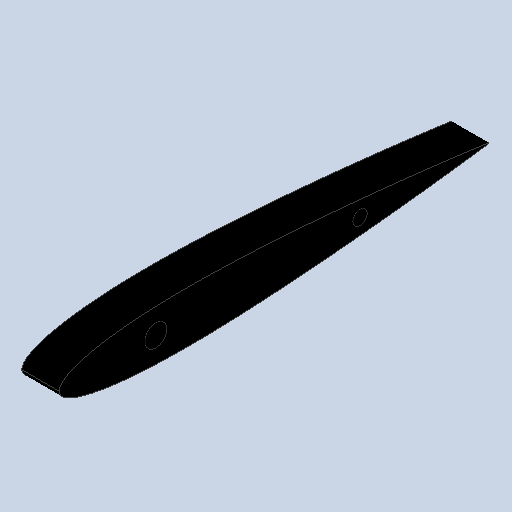
# Autodesk Inventor part: 6P-009
Saved by Autodesk Inventor 2025.2 (Build 292293000, 293)
## iProperties
Category: <PART CATAGORY>
Created: 2024-11-15
Part Number: 6P-009
Material: Poplar
Document SubType Name: Modeling
Designer: lachl
Density: 0.448 g/cm^3
Appearance: Default
Mass: 2.73512 g
Surface Area: 51.8943 cm^2
Volume: 6.10518 cm^3
Title: <TITLE>
Author: lachl
Revision Number: 1
Autodesk Inventor part; units mm, degrees
ref_plane "YZ Plane" through (0, 0, 0) normal (1, 0, 0) x (0, 1, 0)
ref_plane "XZ Plane" through (0, 0, 0) normal (0, 1, 0) x (-1, 0, 0)
ref_plane "XY Plane" through (0, 0, 0) normal (0, 0, 1) x (1, 0, 0)
sketch "Sketch9" plane through (0, 0, 0) normal (1, 0, 0) x (0, 1, 0)
  line L0 (0, 0) -> (0.6838, -0.0937) construction
  line L1 (0.6838, -0.0937) -> (1.3528, -0.3746) construction
  line L2 (1.3528, -0.3746) -> (2.0064, -0.8421) construction
  line L3 (2.0064, -0.8421) -> (2.6435, -1.495) construction
  line L4 (2.6435, -1.495) -> (3.263, -2.3319) construction
  line L5 (3.263, -2.3319) -> (3.8633, -3.3508) construction
  line L6 (3.8633, -3.3508) -> (4.4431, -4.5492) construction
  line L7 (4.4431, -4.5492) -> (5.0005, -5.9245) construction
  line L8 (5.0005, -5.9245) -> (5.5339, -7.4733) construction
  line L9 (5.5339, -7.4733) -> (6.0414, -9.1922) construction
  line L10 (6.0414, -9.1922) -> (6.5213, -11.0769) construction
  line L11 (6.5213, -11.0769) -> (6.9717, -13.1233) construction
  line L12 (6.9717, -13.1233) -> (7.3908, -15.3264) construction
  line L13 (7.3908, -15.3264) -> (7.7773, -17.6811) construction
  line L14 (7.7773, -17.6811) -> (8.1295, -20.182) construction
  line L15 (8.1295, -20.182) -> (8.4463, -22.8232) construction
  line L16 (8.4463, -22.8232) -> (8.7266, -25.5985) construction
  line L17 (8.7266, -25.5985) -> (8.9696, -28.5014) construction
  line L18 (8.9696, -28.5014) -> (9.1748, -31.5252) construction
  line L19 (9.1748, -31.5252) -> (9.3419, -34.6628) construction
  line L20 (9.3419, -34.6628) -> (9.4708, -37.9069) construction
  line L21 (9.4708, -37.9069) -> (9.5619, -41.2498) construction
  line L22 (9.5619, -41.2498) -> (9.6156, -44.6839) construction
  line L23 (9.6156, -44.6839) -> (9.6156, -48.201) construction
  line L24 (9.6156, -48.201) -> (9.6156, -51.793) construction
  line L25 (9.6156, -51.793) -> (9.5617, -55.4514) construction
  line L26 (9.5617, -55.4514) -> (9.4762, -59.1677) construction
  line L27 (9.4762, -59.1677) -> (9.3595, -62.9333) construction
  line L28 (9.3595, -62.9333) -> (9.2132, -66.7394) construction
  line L29 (9.2132, -66.7394) -> (9.0394, -70.5769) construction
  line L30 (9.0394, -70.5769) -> (8.8398, -74.4371) construction
  line L31 (8.8398, -74.4371) -> (8.6167, -78.3109) construction
  line L32 (8.6167, -78.3109) -> (8.372, -82.1891) construction
  line L33 (8.372, -82.1891) -> (8.1078, -86.0629) construction
  line L34 (8.1078, -86.0629) -> (7.8263, -89.9231) construction
  line L35 (7.8263, -89.9231) -> (7.5294, -93.7607) construction
  line L36 (7.5294, -93.7607) -> (7.2193, -97.5667) construction
  line L37 (7.2193, -97.5667) -> (6.8979, -101.3323) construction
  line L38 (6.8979, -101.3323) -> (6.5672, -105.0486) construction
  line L39 (6.5672, -105.0486) -> (6.2291, -108.7071) construction
  line L40 (6.2291, -108.7071) -> (5.8855, -112.299) construction
  line L41 (5.8855, -112.299) -> (5.5382, -115.8161) construction
  line L42 (5.5382, -115.8161) -> (5.1889, -119.2502) construction
  line L43 (5.1889, -119.2502) -> (4.8393, -122.5931) construction
  line L44 (4.8393, -122.5931) -> (4.4912, -125.8372) construction
  line L45 (4.4912, -125.8372) -> (4.1463, -128.9748) construction
  line L46 (4.1463, -128.9748) -> (3.8061, -131.9986) construction
  line L47 (3.8061, -131.9986) -> (3.4724, -134.9015) construction
  line L48 (3.4724, -134.9015) -> (3.1466, -137.6768) construction
  line L49 (3.1466, -137.6768) -> (2.8305, -140.318) construction
  line L50 (2.8305, -140.318) -> (2.5255, -142.8189) construction
  line L51 (2.5255, -142.8189) -> (2.2332, -145.1736) construction
  line L52 (2.2332, -145.1736) -> (1.9553, -147.3767) construction
  line L53 (1.9553, -147.3767) -> (1.693, -149.4231) construction
  line L54 (1.693, -149.4231) -> (1.448, -151.3078) construction
  line L55 (1.448, -151.3078) -> (1.2215, -153.0267) construction
  line L56 (1.2215, -153.0267) -> (1.015, -154.5755) construction
  line L57 (1.015, -154.5755) -> (0.8295, -155.9508) construction
  line L58 (0.8295, -155.9508) -> (0.6664, -157.1492) construction
  line L59 (0.6664, -157.1492) -> (0.5265, -158.1681) construction
  line L60 (0.5265, -158.1681) -> (0.4108, -159.0049) construction
  line L61 (0.4108, -159.0049) -> (0.32, -159.6579) construction
  line L62 (0.32, -159.6579) -> (0.2547, -160.1254) construction
  line L63 (0.2547, -160.1254) -> (0.2154, -160.4063) construction
  line L64 (0.2154, -160.4063) -> (0.2022, -160.5) construction
  line L65 (0.2022, -160.5) -> (0, -161.463) construction
  line L66 (0, -161.463) -> (-0.2022, -160.5) construction
  line L67 (-0.2022, -160.5) -> (-0.2154, -160.4063) construction
  line L68 (-0.2154, -160.4063) -> (-0.2547, -160.1254) construction
  line L69 (-0.2547, -160.1254) -> (-0.32, -159.6579) construction
  line L70 (-0.32, -159.6579) -> (-0.4108, -159.0049) construction
  line L71 (-0.4108, -159.0049) -> (-0.5265, -158.1681) construction
  line L72 (-0.5265, -158.1681) -> (-0.6664, -157.1492) construction
  line L73 (-0.6664, -157.1492) -> (-0.8295, -155.9508) construction
  line L74 (-0.8295, -155.9508) -> (-1.015, -154.5755) construction
  line L75 (-1.015, -154.5755) -> (-1.2215, -153.0267) construction
  line L76 (-1.2215, -153.0267) -> (-1.448, -151.3078) construction
  line L77 (-1.448, -151.3078) -> (-1.693, -149.4231) construction
  line L78 (-1.693, -149.4231) -> (-1.9553, -147.3767) construction
  line L79 (-1.9553, -147.3767) -> (-2.2332, -145.1736) construction
  line L80 (-2.2332, -145.1736) -> (-2.5255, -142.8189) construction
  line L81 (-2.5255, -142.8189) -> (-2.8305, -140.318) construction
  line L82 (-2.8305, -140.318) -> (-3.1466, -137.6768) construction
  line L83 (-3.1466, -137.6768) -> (-3.4724, -134.9015) construction
  line L84 (-3.4724, -134.9015) -> (-3.8061, -131.9986) construction
  line L85 (-3.8061, -131.9986) -> (-4.1463, -128.9748) construction
  line L86 (-4.1463, -128.9748) -> (-4.4912, -125.8372) construction
  line L87 (-4.4912, -125.8372) -> (-4.8393, -122.5931) construction
  line L88 (-4.8393, -122.5931) -> (-5.1889, -119.2502) construction
  line L89 (-5.1889, -119.2502) -> (-5.5382, -115.8161) construction
  line L90 (-5.5382, -115.8161) -> (-5.8855, -112.299) construction
  line L91 (-5.8855, -112.299) -> (-6.2291, -108.7071) construction
  line L92 (-6.2291, -108.7071) -> (-6.5672, -105.0486) construction
  line L93 (-6.5672, -105.0486) -> (-6.8979, -101.3323) construction
  line L94 (-6.8979, -101.3323) -> (-7.2193, -97.5667) construction
  line L95 (-7.2193, -97.5667) -> (-7.5294, -93.7607) construction
  line L96 (-7.5294, -93.7607) -> (-7.8263, -89.9231) construction
  line L97 (-7.8263, -89.9231) -> (-8.1078, -86.0629) construction
  line L98 (-8.1078, -86.0629) -> (-8.372, -82.1891) construction
  line L99 (-8.372, -82.1891) -> (-8.6167, -78.3109) construction
  line L100 (-8.6167, -78.3109) -> (-8.8398, -74.4371) construction
  line L101 (-8.8398, -74.4371) -> (-9.0394, -70.5769) construction
  line L102 (-9.0394, -70.5769) -> (-9.2132, -66.7394) construction
  line L103 (-9.2132, -66.7394) -> (-9.3595, -62.9333) construction
  line L104 (-9.3595, -62.9333) -> (-9.4762, -59.1677) construction
  line L105 (-9.4762, -59.1677) -> (-9.5617, -55.4514) construction
  line L106 (-9.5617, -55.4514) -> (-9.6144, -51.793) construction
  line L107 (-9.6144, -51.793) -> (-9.6144, -48.201) construction
  line L108 (-9.6144, -48.201) -> (-9.6144, -44.6839) construction
  line L109 (-9.6144, -44.6839) -> (-9.5619, -41.2498) construction
  line L110 (-9.5619, -41.2498) -> (-9.4708, -37.9069) construction
  line L111 (-9.4708, -37.9069) -> (-9.3419, -34.6628) construction
  line L112 (-9.3419, -34.6628) -> (-9.1748, -31.5252) construction
  line L113 (-9.1748, -31.5252) -> (-8.9696, -28.5014) construction
  line L114 (-8.9696, -28.5014) -> (-8.7266, -25.5985) construction
  line L115 (-8.7266, -25.5985) -> (-8.4463, -22.8232) construction
  line L116 (-8.4463, -22.8232) -> (-8.1295, -20.182) construction
  line L117 (-8.1295, -20.182) -> (-7.7773, -17.6811) construction
  line L118 (-7.7773, -17.6811) -> (-7.3908, -15.3264) construction
  line L119 (-7.3908, -15.3264) -> (-6.9717, -13.1233) construction
  line L120 (-6.9717, -13.1233) -> (-6.5213, -11.0769) construction
  line L121 (-6.5213, -11.0769) -> (-6.0414, -9.1922) construction
  line L122 (-6.0414, -9.1922) -> (-5.5339, -7.4733) construction
  line L123 (-5.5339, -7.4733) -> (-5.0005, -5.9245) construction
  line L124 (-5.0005, -5.9245) -> (-4.4431, -4.5492) construction
  line L125 (-4.4431, -4.5492) -> (-3.8633, -3.3508) construction
  line L126 (-3.8633, -3.3508) -> (-3.263, -2.3319) construction
  line L127 (-3.263, -2.3319) -> (-2.6435, -1.495) construction
  line L128 (-2.6435, -1.495) -> (-2.0064, -0.8421) construction
  line L129 (-2.0064, -0.8421) -> (-1.3528, -0.3746) construction
  line L130 (-1.3528, -0.3746) -> (-0.6838, -0.0937) construction
  line L131 (-0.6838, -0.0937) -> (0, 0) construction
  spline S0 degree 4 poles (0, 0) (0.6838, -0.0937) (1.3528, -0.3746) (2.0064, -0.8421) (2.6435, -1.495) (3.263, -2.3319) (3.8633, -3.3508) (4.4431, -4.5492) (5.0005, -5.9245) (5.5339, -7.4733) (6.0414, -9.1922) (6.5213, -11.0769) (6.9717, -13.1233) (7.3908, -15.3264) (7.7773, -17.6811) (8.1295, -20.182) (8.4463, -22.8232) (8.7266, -25.5985) (8.9696, -28.5014) (9.1748, -31.5252) (9.3419, -34.6628) (9.4708, -37.9069) (9.5619, -41.2498) (9.6156, -44.6839) (9.6156, -48.201) (9.6156, -51.793) (9.5617, -55.4514) (9.4762, -59.1677) (9.3595, -62.9333) (9.2132, -66.7394) (9.0394, -70.5769) (8.8398, -74.4371) (8.6167, -78.3109) (8.372, -82.1891) (8.1078, -86.0629) (7.8263, -89.9231) (7.5294, -93.7607) (7.2193, -97.5667) (6.8979, -101.3323) (6.5672, -105.0486) (6.2291, -108.7071) (5.8855, -112.299) (5.5382, -115.8161) (5.1889, -119.2502) (4.8393, -122.5931) (4.4912, -125.8372) (4.1463, -128.9748) (3.8061, -131.9986) (3.4724, -134.9015) (3.1466, -137.6768) (2.8305, -140.318) (2.5255, -142.8189) (2.2332, -145.1736) (1.9553, -147.3767) (1.693, -149.4231) (1.448, -151.3078) (1.2215, -153.0267) (1.015, -154.5755) (0.8295, -155.9508) (0.6664, -157.1492) (0.5265, -158.1681) (0.4108, -159.0049) (0.32, -159.6579) (0.2547, -160.1254) (0.2154, -160.4063) (0.2022, -160.5) (0, -161.463) (-0.2022, -160.5) (-0.2154, -160.4063) (-0.2547, -160.1254) (-0.32, -159.6579) (-0.4108, -159.0049) (-0.5265, -158.1681) (-0.6664, -157.1492) (-0.8295, -155.9508) (-1.015, -154.5755) (-1.2215, -153.0267) (-1.448, -151.3078) (-1.693, -149.4231) (-1.9553, -147.3767) (-2.2332, -145.1736) (-2.5255, -142.8189) (-2.8305, -140.318) (-3.1466, -137.6768) (-3.4724, -134.9015) (-3.8061, -131.9986) (-4.1463, -128.9748) (-4.4912, -125.8372) (-4.8393, -122.5931) (-5.1889, -119.2502) (-5.5382, -115.8161) (-5.8855, -112.299) (-6.2291, -108.7071) (-6.5672, -105.0486) (-6.8979, -101.3323) (-7.2193, -97.5667) (-7.5294, -93.7607) (-7.8263, -89.9231) (-8.1078, -86.0629) (-8.372, -82.1891) (-8.6167, -78.3109) (-8.8398, -74.4371) (-9.0394, -70.5769) (-9.2132, -66.7394) (-9.3595, -62.9333) (-9.4762, -59.1677) (-9.5617, -55.4514) (-9.6144, -51.793) (-9.6144, -48.201) (-9.6144, -44.6839) (-9.5619, -41.2498) (-9.4708, -37.9069) (-9.3419, -34.6628) (-9.1748, -31.5252) (-8.9696, -28.5014) (-8.7266, -25.5985) (-8.4463, -22.8232) (-8.1295, -20.182) (-7.7773, -17.6811) (-7.3908, -15.3264) (-6.9717, -13.1233) (-6.5213, -11.0769) (-6.0414, -9.1922) (-5.5339, -7.4733) (-5.0005, -5.9245) (-4.4431, -4.5492) (-3.8633, -3.3508) (-3.263, -2.3319) (-2.6435, -1.495) (-2.0064, -0.8421) (-1.3528, -0.3746) (-0.6838, -0.0937) (0, 0) knots 1 1 1 1 1 2 3 4 5 6 7 8 9 10 11 12 13 14 15 16 17 18 19 20 21 22 23 24 25 26 27 28 29 30 31 32 33 34 35 36 37 38 39 40 41 42 43 44 45 46 47 48 49 50 51 52 53 54 55 56 57 58 59 60 61 62 63 64 65 66 67 68 69 70 71 72 73 74 75 76 77 78 79 80 81 82 83 84 85 86 87 88 89 90 91 92 93 94 95 96 97 98 99 100 101 102 103 104 105 106 107 108 109 110 111 112 113 114 115 116 117 118 119 120 121 122 123 124 125 126 127 128 129 130 130 130 130 130
  constraints: 130 coincident, 4 vertical, 1 other
extrude "Extrusion3" add sketch "Sketch9" along normal blind 14
sketch "Sketch10" plane through (14, 0, 0) normal (1, 0, 0) x (0, 0, -1)
  circle A0 centre (36.25, 0) radius 4.05
  point P0 (0, 0)
  dimension "d88" = 8.1
  dimension "d89" = 36.25
  constraints: 1 centre point
  measures "d88" diameter of A0
  measures "d89" distance of A0.centre point (0, 0)
extrude "Extrusion4" cut sketch "Sketch10" against normal blind 15
sketch "Sketch11" plane through (14, 0, 0) normal (1, 0, 0) x (0, 0, -1)
  circle A0 centre (112.7, 0) radius 2.65
  point P0 (0, 0)
  dimension "d93" = 5.3
  dimension "d94" = 112.7
  constraints: 1 centre point, 1 horizontal alignment
  measures "d93" diameter of A0
  measures "d94" distance of point (0, 0) A0.centre
extrude "Extrusion5" cut sketch "Sketch11" against normal blind 5
body "Solid2"
